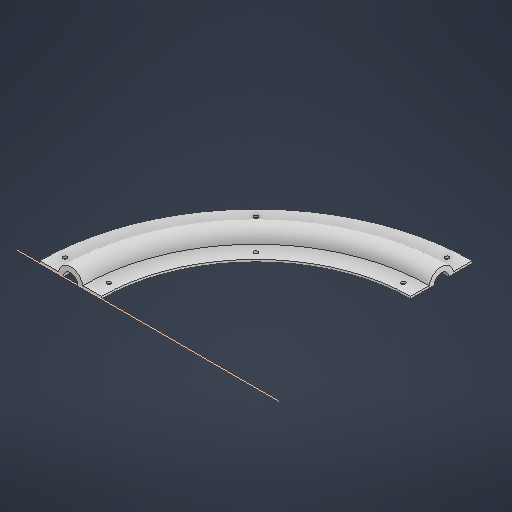
# Autodesk Inventor part: ph-l_mk1
Saved by Autodesk Inventor 2026.1 (Build 301233000, 233)
## iProperties
Created: 2025-11-03
Part Number: ph-l_mk1
Material: Generisch
Document SubType Name: Modeling
Designer: RunHD
Density: 1 g/cm^3
Appearance: Vorgabe
Author: RunHD
Autodesk Inventor part; units mm, degrees
ref_plane "YZ Plane" through (0, 0, 0) normal (1, 0, 0) x (0, 1, 0)
ref_plane "XZ Plane" through (0, 0, 0) normal (0, 1, 0) x (-1, 0, 0)
ref_plane "XY Plane" through (0, 0, 0) normal (0, 0, 1) x (1, 0, 0)
sketch "Skizze1" plane through (0, 0, 0) normal (0, 0, 1) x (1, 0, 0)
  arc A0 (0, 180) -> (-180, 0) centre (0, 0) ccw
  line L0 (-260.7351, 0) -> (43.4558, 0) projected
  line L1 (0, -43.4558) -> (0, 260.7351) projected
  dimension "d0" = 180
  dimension "d1" = 90
  constraints: 2 point on circle, 1 centre point, 1 coincident, 1 point on line
  measures "d0" radius of A0
sketch "Skizze2" plane through (0, 0, 0) normal (0, 1, 0) x (-1, 0, 0)
  line L0 (0, -42) -> (0, 42) projected
  circle A0 centre (180, 0) radius 7
  line L1 (252, 0) -> (-42, 0) projected
  circle A1 centre (180, 0) radius 12
  line L2 (191.9553, 0) -> (168, 0)
  line L3 (173, 0) -> (160, 0)
  line L4 (173, 2) -> (173, 0)
  line L5 (187, 0) -> (200, 0)
  line L6 (187, 2) -> (187, 0)
  circle A2 centre (180, 0) radius 30
  line L7 (187, 2) -> (209.9333, 2)
  line L8 (173, 2) -> (150.0667, 2)
  point P0 (0, 0)
  point P1 (173, 0)
  point P2 (168, 0)
  point P3 (192, 0)
  point P4 (191.8322, 2)
  point P5 (168.1678, 2)
  point P6 (150, 0)
  point P7 (210, 0)
  dimension "d5" = 24
  dimension "d3" = 180
  dimension "d4" = 14
  dimension "d16" = 60
  dimension "d17" = 2
  dimension "d18" = 23
  dimension "d19" = 7
  constraints: 14 end point, 5 point on line, 4 point on circle, 3 horizontal, 2 centre point, 1 collinear, 5 other
  measures "d3" distance from line of L0 A0.centre
  measures "d4" diameter of A0
  measures "d16" diameter of A2
  measures "d17" distance between parallel lines of L3 L8
  measures "d18" distance edge to line of A2 L4
  measures "d19" distance from line of A2.centre L6
sweep "Sweeping1" add profiles "Skizze2" path "Skizze1" path curves A0 contours L6 L7 A1 L1 | A0 L4 L8 A1 L7 L6 | L1 A1 L8 L4 | L1 A2 L8 A1 | A1 L7 A2 L1
sketch "Skizze7" plane through (-168.1678, 0, 2) normal (0, 0, 1) x (1, 0, 0)
  line L0 (18.1678, 0) -> (18.1678, -3) projected
  line L1 (0, 0) -> (18.1011, 0) projected
  line L2 (168.1678, 150) -> (171.1678, 150) projected
  line L3 (168.1678, 168.1678) -> (168.1678, 150.0667) projected
  line L4 (168.1678, 210) -> (171.1678, 210) projected
  arc A0 (168.1678, 150.0667) -> (18.1011, 0) centre (168.1678, 0) ccw projected
  circle A1 centre (168.1678, 0) radius 168 projected
  line L5 (-41.8322, 0) -> (-41.8322, -3) projected
  point P0 (10.1678, 15)
  point P1 (56.0828, 112.085)
  point P2 (153.1678, 158)
  dimension "d36" = 8
  dimension "d37" = 15
  dimension "d38" = 8
  dimension "d39" = 15
  dimension "d41" = 97.915
  dimension "d42" = 97.915
  measures "d36" distance from line of L0 point (10.168, 15)
  measures "d37" distance from line of L1 point (10.168, 15)
  measures "d38" distance from line of L2 point (153.168, 158)
  measures "d39" distance from line of L3 point (153.168, 158)
  measures "d41" distance from line of point (56.083, 112.085) L4
  measures "d42" distance from line of point (56.083, 112.085) L5
hole "Bohrung1" at (-158, 15, 2) at (-112.085, 112.085, 2) at (-15, 158, 2) direction (0, 0, -1) diameter 4 depth 8
sketch "Skizze8" plane through (-209.9333, 0, 2) normal (0, 0, 1) x (1, 0, 0)
  line L0 (-0.0667, 0) -> (-0.0667, -3) projected
  line L1 (0, 0) -> (18.1011, 0) projected
  line L2 (209.9333, 209.9333) -> (209.9333, 191.8322) projected
  line L3 (209.9333, 210) -> (212.9333, 210) projected
  arc A0 (209.9333, 168.1678) -> (41.7654, 0) centre (209.9333, 0) ccw projected
  circle A1 centre (209.9333, 0) radius 200.8827
  point P0 (209.9333, 0)
  point P1 (9.6113, 15)
  point P2 (67.8861, 142.044)
  point P3 (194.9333, 200.3219)
  dimension "d51" = 15
  dimension "d52" = 15
  dimension "d54" = 142.044
  dimension "d59" = 401.7655
  dimension "d60" = 142.0471
  constraints: 3 point on circle, 1 centre point, 1 coincident
  measures "d51" distance from line of L1 A1.end
  measures "d52" distance from line of L2 A1.start
  measures "d54" distance from line of point (67.886, 142.044) L1
  measures "d59" diameter of A1
  measures "d60" distance from line of L2 point (67.886, 142.044)
hole "Bohrung3" at (-200.3219, 15, 2) at (-142.0471, 142.044, 2) at (-15, 200.3219, 2) direction (0, 0, -1) diameter 4 depth 8
